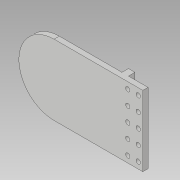
# Autodesk Inventor part: dynamixel_pro_frame_part2
Saved by Autodesk Inventor 2017 (Build 210142000, 142)
## iProperties
Part Number: dynamixel_pro_frame_part2
Material: Aluminium 6061
Document SubType Name: Modeling
Designer: Max
Density: 2.7 g/cm^3
Appearance: Vorgabe
Author: Max
Autodesk Inventor part; units mm, degrees
ref_plane "YZ Plane" through (0, 0, 0) normal (1, 0, 0) x (0, 1, 0)
ref_plane "XZ Plane" through (0, 0, 0) normal (0, 1, 0) x (-1, 0, 0)
ref_plane "XY Plane" through (0, 0, 0) normal (0, 0, 1) x (1, 0, 0)
sketch "Skizze1" plane through (0, 0, 0) normal (0, 1, 0) x (-1, 0, 0)
  line L0 (-50, 27) -> (50, 27)
  line L1 (50, 27) -> (50, -27) construction
  line L2 (50, -27) -> (-50, -27)
  line L3 (-50, -27) -> (-50, 27)
  line L4 (-50, 27) -> (50, -27) construction
  line L5 (50, 27) -> (-50, -27) construction
  line L6 (0, 0) -> (66.4326, 0) construction
  arc A0 (18, -27) -> (18, 27) centre (18, 0) ccw
  dimension "d0" = 54
  dimension "d1" = 100
  dimension "d12" = 68
  dimension "d13" = 90
  constraints: 14 end point, 3 point on line, 2 horizontal, 2 midpoint, 2 parallel, 2 point on circle, 1 centre point, 1 perpendicular
  measures "d0" distance of L2.end L0.start
  measures "d1" distance of L1.end L2.end
  measures "d12" distance from line of A0.centre L3
extrude "Extrusion1" add sketch "Skizze1" along normal blind 4
sketch "Skizze3" plane through (0, 4, 0) normal (0, 1, 0) x (1, 0, 0)
  circle A0 centre (-18, 0) radius 6
  line L0 (0, 0) -> (-17.1865, 0) construction
  line L1 (50, -27) -> (50, 27) construction
  line L2 (-18, -27) -> (50, -27) projected
  line L3 (50, -27) -> (50, 27) construction
  line L4 (50, 27) -> (-18, 27) construction
  line L5 (-18, -27) -> (50, -27) construction
  line L6 (50, 27) -> (-18, 27) construction
  arc A1 (-18, 27) -> (-18, -27) centre (-18, 0) ccw projected
  point P0 (-50, -27)
  point P1 (-50, 27)
  dimension "d8" = 12
  dimension "d9" = 68
  constraints: 2 end point, 1 centre point, 1 horizontal, 1 point on line
  measures "d8" diameter of A0
  measures "d9" distance from line of L1 A0.centre
extrude "Extrusion3" [suppressed]
sketch "Skizze5" plane through (0, 4, 0) normal (0, 1, 0) x (1, 0, 0)
  line L0 (-18, -27) -> (50, -27) projected
  line L1 (50, -27) -> (50, 27) projected
  line L2 (50, 27) -> (-18, 27) projected
  arc A0 (-18, 27) -> (-18, -27) centre (-18, 0) ccw projected
  line L3 (35, -27) -> (30, -27)
  line L4 (30, -27) -> (30, 27)
  line L5 (30, 27) -> (35, 27)
  line L6 (35, 27) -> (35, -27)
  point P0 (0, 0)
  dimension "d14" = 15
  dimension "d15" = 5
  constraints: 8 end point, 2 parallel, 2 point on line, 1 horizontal, 1 perpendicular
  measures "d14" distance between parallel lines of L6 L1
  measures "d15" distance between parallel lines of L4 L6
extrude "Extrusion4" add sketch "Skizze5" along normal blind 5 contours L4 L2 L6 L0
sketch "Skizze6" plane through (0, 4, 0) normal (0, 1, 0) x (1, 0, 0)
  line L0 (35, 27) -> (35, -27) projected
  line L1 (35, -27) -> (50, -27) projected
  line L2 (50, -27) -> (50, 27) projected
  line L3 (50, 27) -> (35, 27) projected
  line L4 (0, 0) -> (67.4565, 0) construction
  point P0 (46.5, 0)
  dimension "d18" = 3.5
  constraints: 2 end point, 1 horizontal, 1 point on line
  measures "d18" distance from line of point (46.5, 0) L2
hole "Bohrung1" at (46.5, 4, 0) direction (0, -1, 0) diameter 3.4 end through all clearance for "Inbusschraube ISO 4762" size "M3" standard "ISO"
pattern_linear "Rechteckige Anordnung1" count 5 spacing 11 along (0, 0, -1) count 2 spacing 8 along (-1, 0, 0) of "Bohrung1" first direction both ways yes
sketch "Skizze7" plane through (0, 0, 0) normal (0, -1, 0) x (1, 0, 0)
  circle A0 centre (-18, 0) radius 6 projected
  circle A1 centre (-18, 0) radius 10 construction
  line L0 (-18, -12.7159) -> (-18, 15.8855)
  line L1 (-33.0539, 0) -> (-6.7164, 0)
  point P0 (0, 0)
  point P1 (-18, -10)
  point P2 (-28, 0)
  point P3 (-18, 10)
  point P4 (-8, 0)
  dimension "d32" = 20
  constraints: 6 point on line, 4 end point, 4 point on circle, 1 centre point, 1 coincident, 1 horizontal, 1 vertical
  measures "d32" diameter of A1
hole "Bohrung2" [suppressed]
sketch "Skizze8" plane through (0, 4, 0) normal (0, 1, 0) x (1, 0, 0)
  arc A0 (-18, 27) -> (-18, -27) centre (-18, 0) ccw projected
  circle A1 centre (-18, 0) radius 6
  circle A2 centre (-18, 0) radius 4
  point P0 (0, 0)
  dimension "d40" = 12
  dimension "d43" = 8
  constraints: 2 centre point, 2 coincident
  measures "d40" diameter of A1
  measures "d43" diameter of A2
extrude "Extrusion5" add sketch "Skizze8" along normal blind 3 contours A1 | A2
extrude "Extrusion6" add sketch "Skizze8" along normal blind 10 contours A2
